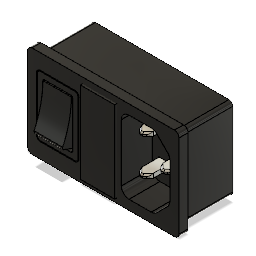
Power Receptacle (Jameco IEC-GS-1-100) v3 (Autodesk Fusion 360 design; units mm, degrees)
Autodesk Fusion 360 part; units mm, degrees
note: some values were not read from the file. Chosen so that the rebuilt part matches the saved one: which face or edge a step refers to.
sketch "Sketch1" plane through (0, 0, 0) normal (0, 0, 1) x (1, 0, 0)
  line L0 (0, 0) -> (49.9872, 0)
  line L1 (49.9872, 0) -> (49.9872, 30.48)
  line L2 (49.9872, 30.48) -> (0, 30.48)
  line L3 (0, 30.48) -> (0, 0)
  dimension "d1" = 30.48
  dimension "d2" = 49.9872
  measures "d1" distance of L0.start
  measures "d2" distance of L0.start
extrude "Extrude1" add sketch "Sketch1" against normal blind 2.9972 makes body 1
fillet "Fillet1" radius 1.4986 4 edges at (49.9872, 30.48, -1.4986) (0, 30.48, -1.4986) (0, 0, -1.4986) (49.9872, 0, -1.4986) on bodies 1
sketch "Sketch2" plane through (0, 0, -2.9972) normal (0, 0, -1) x (-1, 0, 0)
  arc A0 (-49.9872, 1.4986) -> (-48.4886, 0) centre (-48.4886, 1.4986) ccw
  line L0 (-48.4886, 0) -> (-1.4986, 0)
  arc A1 (-1.4986, 0) -> (0, 1.4986) centre (-1.4986, 1.4986) ccw
  line L1 (0, 1.4986) -> (0, 28.9814)
  arc A2 (0, 28.9814) -> (-1.4986, 30.48) centre (-1.4986, 28.9814) ccw
  line L2 (-1.4986, 30.48) -> (-48.4886, 30.48)
  arc A3 (-48.4886, 30.48) -> (-49.9872, 28.9814) centre (-48.4886, 28.9814) ccw
  line L3 (-49.9872, 28.9814) -> (-49.9872, 1.4986)
  line L4 (-24.9936, 30.48) -> (-24.9936, 0) construction
  line L5 (0, 15.24) -> (-49.9872, 15.24) construction
  line L6 (-49.9872, 30.48) -> (-49.9872, 0) construction
  line L7 (-49.9872, 0) -> (0, 0) construction
  line L8 (0, 0) -> (0, 30.48) construction
  line L9 (0, 30.48) -> (-49.9872, 30.48) construction
  line L10 (-48.2854, 1.7399) -> (-1.7018, 1.7399)
  line L11 (-1.7018, 1.7399) -> (-1.7018, 28.7401)
  line L12 (-1.7018, 28.7401) -> (-48.2854, 28.7401)
  line L13 (-48.2854, 28.7401) -> (-48.2854, 1.7399)
  line L14 (-48.2854, 28.7401) -> (-48.2854, 30.48) construction
  line L15 (-48.2854, 28.7401) -> (-49.9872, 28.7401) construction
  line L16 (-1.7018, 1.7399) -> (-1.7018, 0) construction
  line L17 (-1.7018, 1.7399) -> (0, 1.7399) construction
  dimension "d6" = 27.0002
  dimension "d7" = 46.5836
  measures "d6" distance of L7.end
  measures "d7" distance of L7.end
extrude "Extrude2" add sketch "Sketch2" along normal blind 16.4846 contours L10 L11 L12 L13 bodies 1
fillet "Fillet2" radius 1.27 4 edges at (48.2854, 28.7401, -11.2395) (1.7018, 28.7401, -11.2395) (1.7018, 1.7399, -11.2395) (48.2854, 1.7399, -11.2395) on bodies 1
sketch "Sketch3" plane through (0, 0, 0) normal (0, 0, 1) x (1, 0, 0)
  arc A0 (48.4886, 0) -> (49.9872, 1.4986) centre (48.4886, 1.4986) ccw
  line L0 (49.9872, 1.4986) -> (49.9872, 28.9814)
  arc A1 (49.9872, 28.9814) -> (48.4886, 30.48) centre (48.4886, 28.9814) ccw
  line L1 (48.4886, 30.48) -> (1.4986, 30.48)
  arc A2 (1.4986, 30.48) -> (0, 28.9814) centre (1.4986, 28.9814) ccw
  line L2 (0, 28.9814) -> (0, 1.4986)
  arc A3 (0, 1.4986) -> (1.4986, 0) centre (1.4986, 1.4986) ccw
  line L3 (1.4986, 0) -> (48.4886, 0)
  line L4 (30.9852, 5.7785) -> (30.9852, 24.7015)
  line L5 (33.5252, 27.2415) -> (40.8551, 27.2415)
  line L6 (42.6511, 26.4976) -> (46.2433, 22.9054)
  line L7 (46.9872, 21.1094) -> (46.9872, 9.3706)
  line L8 (46.2433, 7.5746) -> (42.6511, 3.9824)
  line L9 (40.8551, 3.2385) -> (33.5252, 3.2385)
  arc A4 (33.5252, 27.2415) -> (30.9852, 24.7015) centre (33.5252, 24.7015) ccw
  arc A5 (30.9852, 5.7785) -> (33.5252, 3.2385) centre (33.5252, 5.7785) ccw
  arc A6 (42.6511, 26.4976) -> (40.8551, 27.2415) centre (40.8551, 24.7015) ccw
  arc A7 (46.9872, 21.1094) -> (46.2433, 22.9054) centre (44.4472, 21.1094) ccw
  arc A8 (46.2433, 7.5746) -> (46.9872, 9.3706) centre (44.4472, 9.3706) ccw
  arc A9 (40.8551, 3.2385) -> (42.6511, 3.9824) centre (40.8551, 5.7785) ccw
  line L10 (36.1112, 3.2385) -> (36.1112, 0) construction
  line L11 (37.1901, 27.2415) -> (37.1901, 30.48) construction
  dimension "d11" = 135
  dimension "d12" = 135
  dimension "d13" = 24.003
  dimension "d14" = 16.002
  dimension "d15" = 5.08
  dimension "d16" = 2.54
  dimension "d17" = 2.54
  dimension "d18" = 3
  measures "d11" angle of L8 L9
  measures "d12" angle of L5 L6
  measures "d13" distance of origin
  measures "d14" distance of L4 L7
  measures "d16" radius of A4
  measures "d17" radius of A9
  measures "d18" distance of L0 L7
extrude "Extrude3" cut sketch "Sketch3" against normal blind 10.16 contours L4 L5 L6 L7 L8 L9 A4 A5 A6 A7 A8 A9 bodies 1
sketch "Sketch4" plane through (0, 0, 0) normal (0, 0, 1) x (1, 0, 0)
  line L0 (42.6511, 26.4976) -> (46.2433, 22.9054)
  arc A0 (46.9872, 21.1094) -> (46.2433, 22.9054) centre (44.4472, 21.1094) ccw
  line L1 (46.9872, 21.1094) -> (46.9872, 9.3706)
  arc A1 (46.2433, 7.5746) -> (46.9872, 9.3706) centre (44.4472, 9.3706) ccw
  line L2 (46.2433, 7.5746) -> (42.6511, 3.9824)
  arc A2 (40.8551, 3.2385) -> (42.6511, 3.9824) centre (40.8551, 5.7785) ccw
  line L3 (40.8551, 3.2385) -> (33.5252, 3.2385)
  arc A3 (30.9852, 5.7785) -> (33.5252, 3.2385) centre (33.5252, 5.7785) ccw
  line L4 (30.9852, 5.7785) -> (30.9852, 24.7015)
  arc A4 (33.5252, 27.2415) -> (30.9852, 24.7015) centre (33.5252, 24.7015) ccw
  line L5 (33.5252, 27.2415) -> (40.8551, 27.2415)
  arc A5 (42.6511, 26.4976) -> (40.8551, 27.2415) centre (40.8551, 24.7015) ccw
  arc A6 (48.4886, 0) -> (49.9872, 1.4986) centre (48.4886, 1.4986) ccw
  line L6 (49.9872, 1.4986) -> (49.9872, 28.9814)
  arc A7 (49.9872, 28.9814) -> (48.4886, 30.48) centre (48.4886, 28.9814) ccw
  line L7 (48.4886, 30.48) -> (1.4986, 30.48)
  arc A8 (1.4986, 30.48) -> (0, 28.9814) centre (1.4986, 28.9814) ccw
  line L8 (0, 28.9814) -> (0, 1.4986)
  arc A9 (0, 1.4986) -> (1.4986, 0) centre (1.4986, 1.4986) ccw
  line L9 (1.4986, 0) -> (48.4886, 0)
  line L10 (4.27, 5.08) -> (15.7, 5.08)
  line L11 (16.97, 6.35) -> (16.97, 24.13)
  line L12 (15.7, 25.4) -> (4.27, 25.4)
  line L13 (3, 24.13) -> (3, 6.35)
  line L14 (9.985, 25.4) -> (9.985, 30.48) construction
  line L15 (9.985, 5.08) -> (9.985, 0) construction
  arc A10 (16.97, 24.13) -> (15.7, 25.4) centre (15.7, 24.13) ccw
  arc A11 (15.7, 5.08) -> (16.97, 6.35) centre (15.7, 6.35) ccw
  arc A12 (3, 6.35) -> (4.27, 5.08) centre (4.27, 6.35) ccw
  arc A13 (4.27, 25.4) -> (3, 24.13) centre (4.27, 24.13) ccw
  dimension "d21" = 20.32
  dimension "d22" = 13.97
  dimension "d23" = 3
  dimension "d24" = 1.27
  dimension "d25" = 1.27
  measures "d23" distance of L8 L13
  measures "d24" radius of A10
  measures "d25" radius of A13
extrude "Extrude4" cut sketch "Sketch4" against normal blind 2.9972 contours L10 L11 L12 L13 A10 A11 A12 A13 bodies 1
sketch "Sketch5" plane through (0, 0, -2.9972) normal (0, 0, 1) x (1, 0, 0)
  arc A0 (4.27, 25.4) -> (3, 24.13) centre (4.27, 24.13) ccw
  line L0 (3, 24.13) -> (3, 6.35)
  arc A1 (3, 6.35) -> (4.27, 5.08) centre (4.27, 6.35) ccw
  line L1 (4.27, 5.08) -> (15.7, 5.08)
  arc A2 (15.7, 5.08) -> (16.97, 6.35) centre (15.7, 6.35) ccw
  line L2 (16.97, 6.35) -> (16.97, 24.13)
  arc A3 (16.97, 24.13) -> (15.7, 25.4) centre (15.7, 24.13) ccw
  line L3 (15.7, 25.4) -> (4.27, 25.4)
  line L4 (15.7, 6.35) -> (15.7, 24.13)
  line L5 (15.7, 24.13) -> (4.27, 24.13)
  line L6 (4.27, 24.13) -> (4.27, 6.35)
  line L7 (4.27, 6.35) -> (15.7, 6.35)
  dimension "d28" = 1.27
  measures "d28" distance of L2
extrude "Extrude5" cut sketch "Sketch5" against normal blind 50.8 contours L4 L5 L6 L7 bodies 1
sketch "Sketch6" plane through (0, 0, -2.9972) normal (0, 0, 1) x (1, 0, 0)
  line L0 (15.7, 24.13) -> (15.7, 6.35)
  line L1 (15.7, 6.35) -> (4.27, 6.35)
  line L2 (4.27, 6.35) -> (4.27, 24.13)
  line L3 (4.27, 24.13) -> (15.7, 24.13)
  arc A0 (4.27, 25.4) -> (3, 24.13) centre (4.27, 24.13) ccw
  line L4 (3, 24.13) -> (3, 6.35)
  arc A1 (3, 6.35) -> (4.27, 5.08) centre (4.27, 6.35) ccw
  line L5 (4.27, 5.08) -> (15.7, 5.08)
  arc A2 (15.7, 5.08) -> (16.97, 6.35) centre (15.7, 6.35) ccw
  line L6 (16.97, 6.35) -> (16.97, 24.13)
  arc A3 (16.97, 24.13) -> (15.7, 25.4) centre (15.7, 24.13) ccw
  line L7 (15.7, 25.4) -> (4.27, 25.4)
  line L8 (4.27, 5.334) -> (15.7, 5.334)
  arc A4 (15.7, 5.334) -> (16.716, 6.35) centre (15.7, 6.35) ccw
  line L9 (16.716, 6.35) -> (16.716, 24.13)
  arc A5 (16.716, 24.13) -> (15.7, 25.146) centre (15.7, 24.13) ccw
  line L10 (15.7, 25.146) -> (4.27, 25.146)
  arc A6 (4.27, 25.146) -> (3.254, 24.13) centre (4.27, 24.13) ccw
  line L11 (3.254, 24.13) -> (3.254, 6.35)
  arc A7 (3.254, 6.35) -> (4.27, 5.334) centre (4.27, 6.35) ccw
  line L12 (14.938, 7.112) -> (5.032, 7.112)
  line L13 (5.032, 7.112) -> (5.032, 23.368)
  line L14 (5.032, 23.368) -> (14.938, 23.368)
  line L15 (14.938, 23.368) -> (14.938, 7.112)
  dimension "d32" = 0.254
  dimension "d33" = 0.762
  measures "d32" distance of L5
  measures "d33" distance of L1
extrude "Extrude6" add sketch "Sketch6" along normal up to surface (2.9972 mm away) separate body contours L0 L1 L2 L3 | L8 A4 L9 A5 L10 A6 L11 A7 makes body 2
fillet "Fillet3" radius 0.635 4 edges at (5.032, 23.368, -1.4986) (14.938, 23.368, -1.4986) (5.032, 7.112, -1.4986) (14.938, 7.112, -1.4986) on bodies 2
sketch "Sketch7" plane through (0, 0, -2.9972) normal (0, 0, -1) x (-1, 0, 0)
  arc A0 (-14.938, 7.747) -> (-14.303, 7.112) centre (-14.303, 7.747) ccw
  line L0 (-14.938, 7.747) -> (-14.938, 22.733)
  arc A1 (-14.303, 23.368) -> (-14.938, 22.733) centre (-14.303, 22.733) ccw
  line L1 (-14.303, 23.368) -> (-5.667, 23.368)
  arc A2 (-5.032, 22.733) -> (-5.667, 23.368) centre (-5.667, 22.733) ccw
  line L2 (-5.032, 22.733) -> (-5.032, 7.747)
  arc A3 (-5.667, 7.112) -> (-5.032, 7.747) centre (-5.667, 7.747) ccw
  line L3 (-5.667, 7.112) -> (-14.303, 7.112)
  arc A4 (-4.27, 5.334) -> (-3.254, 6.35) centre (-4.27, 6.35) ccw
  line L4 (-3.254, 6.35) -> (-3.254, 24.13)
  arc A5 (-3.254, 24.13) -> (-4.27, 25.146) centre (-4.27, 24.13) ccw
  line L5 (-4.27, 25.146) -> (-15.7, 25.146)
  arc A6 (-15.7, 25.146) -> (-16.716, 24.13) centre (-15.7, 24.13) ccw
  line L6 (-16.716, 24.13) -> (-16.716, 6.35)
  arc A7 (-16.716, 6.35) -> (-15.7, 5.334) centre (-15.7, 6.35) ccw
  line L7 (-15.7, 5.334) -> (-4.27, 5.334)
  line L8 (-15.1788, 23.6625) -> (-4.7856, 23.6625)
  line L9 (-4.7856, 23.6625) -> (-4.7856, 6.7161)
  line L10 (-4.7856, 6.7161) -> (-15.1788, 6.7161)
  line L11 (-15.1788, 6.7161) -> (-15.1788, 23.6625)
extrude "Extrude7" add sketch "Sketch7" along normal blind 11.43 contours A0 L0 A1 L1 A2 L2 A3 L3 | L8 L9 L10 L11 bodies 2
sketch "Sketch8" plane through (0, 0, -2.9972) normal (0, 0, 1) x (1, 0, 0)
  arc A0 (14.938, 22.733) -> (14.303, 23.368) centre (14.303, 22.733) ccw
  line L0 (14.303, 23.368) -> (5.667, 23.368)
  arc A1 (5.667, 23.368) -> (5.032, 22.733) centre (5.667, 22.733) ccw
  line L1 (5.032, 22.733) -> (5.032, 7.747)
  arc A2 (5.032, 7.747) -> (5.667, 7.112) centre (5.667, 7.747) ccw
  line L2 (5.667, 7.112) -> (14.303, 7.112)
  arc A3 (14.303, 7.112) -> (14.938, 7.747) centre (14.303, 7.747) ccw
  line L3 (14.938, 7.747) -> (14.938, 22.733)
  line L4 (14.684, 7.747) -> (14.684, 22.733)
  arc A4 (14.684, 22.733) -> (14.303, 23.114) centre (14.303, 22.733) ccw
  line L5 (14.303, 23.114) -> (5.667, 23.114)
  arc A5 (5.667, 23.114) -> (5.286, 22.733) centre (5.667, 22.733) ccw
  line L6 (5.286, 22.733) -> (5.286, 7.747)
  arc A6 (5.286, 7.747) -> (5.667, 7.366) centre (5.667, 7.747) ccw
  line L7 (5.667, 7.366) -> (14.303, 7.366)
  arc A7 (14.303, 7.366) -> (14.684, 7.747) centre (14.303, 7.747) ccw
  dimension "d39" = 0.254
  measures "d39" distance of L3
extrude "Extrude8" add sketch "Sketch8" along normal blind 6.35 separate body contours L4 A4 L5 A5 L6 A6 L7 A7 makes body 3
sketch "Sketch9" plane through (5.286, 0, 0) normal (-1, 0, 0) x (0, 0, 1)
  line L0 (-2.9972, 7.747) -> (3.3528, 7.747)
  line L1 (3.3528, 7.747) -> (3.3528, 22.733)
  line L2 (3.3528, 22.733) -> (-2.9972, 22.733)
  line L3 (-2.9972, 7.2231) -> (3.3528, 9.5788)
  arc A0 (0.1778, 23.4401) -> (3.3528, 9.5788) centre (31.7454, 23.3766) ccw
  line L4 (-2.9972, 7.2231) -> (-2.9972, -1.1091)
  line L5 (-2.9972, -1.1091) -> (15.3397, -2.5698)
  line L6 (15.3397, -2.5698) -> (9.4997, 23.1267)
  line L7 (9.4997, 23.1267) -> (0.1778, 23.4401)
  line L8 (-2.9972, 22.733) -> (-2.9972, 7.747)
extrude "Extrude9" cut sketch "Sketch9" against normal blind 20.32 contours L0 L1 L3 | L0 L1 L2 L3 A0 L4 L5 L6 L7 | L1 L2 A0 bodies 3
fillet "Fillet4" radius 0.635 1 edges at (9.985, 9.5788, 3.3528) on bodies 3
sketch "Sketch10" plane through (0, 0, 0) normal (0, 0, 1) x (1, 0, 0)
  line L0 (3, 6.35) -> (3, 24.13)
  arc A0 (4.27, 25.4) -> (3, 24.13) centre (4.27, 24.13) ccw
  line L1 (4.27, 25.4) -> (15.7, 25.4)
  arc A1 (16.97, 24.13) -> (15.7, 25.4) centre (15.7, 24.13) ccw
  line L2 (16.97, 24.13) -> (16.97, 6.35)
  arc A2 (15.7, 5.08) -> (16.97, 6.35) centre (15.7, 6.35) ccw
  line L3 (15.7, 5.08) -> (4.27, 5.08)
  arc A3 (3, 6.35) -> (4.27, 5.08) centre (4.27, 6.35) ccw
  line L4 (42.6511, 26.4976) -> (46.2433, 22.9054)
  arc A4 (46.9872, 21.1094) -> (46.2433, 22.9054) centre (44.4472, 21.1094) ccw
  line L5 (46.9872, 21.1094) -> (46.9872, 9.3706)
  arc A5 (46.2433, 7.5746) -> (46.9872, 9.3706) centre (44.4472, 9.3706) ccw
  line L6 (46.2433, 7.5746) -> (42.6511, 3.9824)
  arc A6 (40.8551, 3.2385) -> (42.6511, 3.9824) centre (40.8551, 5.7785) ccw
  line L7 (40.8551, 3.2385) -> (33.5252, 3.2385)
  arc A7 (30.9852, 5.7785) -> (33.5252, 3.2385) centre (33.5252, 5.7785) ccw
  line L8 (30.9852, 5.7785) -> (30.9852, 24.7015)
  arc A8 (33.5252, 27.2415) -> (30.9852, 24.7015) centre (33.5252, 24.7015) ccw
  line L9 (33.5252, 27.2415) -> (40.8551, 27.2415)
  arc A9 (42.6511, 26.4976) -> (40.8551, 27.2415) centre (40.8551, 24.7015) ccw
  arc A10 (48.4886, 0) -> (49.9872, 1.4986) centre (48.4886, 1.4986) ccw
  line L10 (49.9872, 1.4986) -> (49.9872, 28.9814)
  arc A11 (49.9872, 28.9814) -> (48.4886, 30.48) centre (48.4886, 28.9814) ccw
  line L11 (48.4886, 30.48) -> (1.4986, 30.48)
  arc A12 (1.4986, 30.48) -> (0, 28.9814) centre (1.4986, 28.9814) ccw
  line L12 (0, 28.9814) -> (0, 1.4986)
  arc A13 (0, 1.4986) -> (1.4986, 0) centre (1.4986, 1.4986) ccw
  line L13 (1.4986, 0) -> (48.4886, 0)
  line L14 (19.5925, 27.5743) -> (28.391, 27.5743)
  line L15 (28.391, 27.5743) -> (28.391, 2.7579)
  line L16 (28.391, 2.7579) -> (19.5925, 2.7579)
  line L17 (19.5925, 2.7579) -> (19.5925, 27.5743)
extrude "Extrude10" cut sketch "Sketch10" against normal blind 7.62 contours L14 L15 L16 L17 bodies 1
sketch "Sketch11" plane through (0, 0, 0) normal (0, 0, 1) x (1, 0, 0)
  line L0 (28.391, 27.5743) -> (28.391, 2.7579)
  line L1 (28.391, 2.7579) -> (19.5925, 2.7579)
  line L2 (19.5925, 2.7579) -> (19.5925, 27.5743)
  line L3 (19.5925, 27.5743) -> (28.391, 27.5743)
  line L4 (3, 6.35) -> (3, 24.13)
  arc A0 (4.27, 25.4) -> (3, 24.13) centre (4.27, 24.13) ccw
  line L5 (4.27, 25.4) -> (15.7, 25.4)
  arc A1 (16.97, 24.13) -> (15.7, 25.4) centre (15.7, 24.13) ccw
  line L6 (16.97, 24.13) -> (16.97, 6.35)
  arc A2 (15.7, 5.08) -> (16.97, 6.35) centre (15.7, 6.35) ccw
  line L7 (15.7, 5.08) -> (4.27, 5.08)
  arc A3 (3, 6.35) -> (4.27, 5.08) centre (4.27, 6.35) ccw
  line L8 (42.6511, 26.4976) -> (46.2433, 22.9054)
  arc A4 (46.9872, 21.1094) -> (46.2433, 22.9054) centre (44.4472, 21.1094) ccw
  line L9 (46.9872, 21.1094) -> (46.9872, 9.3706)
  arc A5 (46.2433, 7.5746) -> (46.9872, 9.3706) centre (44.4472, 9.3706) ccw
  line L10 (46.2433, 7.5746) -> (42.6511, 3.9824)
  arc A6 (40.8551, 3.2385) -> (42.6511, 3.9824) centre (40.8551, 5.7785) ccw
  line L11 (40.8551, 3.2385) -> (33.5252, 3.2385)
  arc A7 (30.9852, 5.7785) -> (33.5252, 3.2385) centre (33.5252, 5.7785) ccw
  line L12 (30.9852, 5.7785) -> (30.9852, 24.7015)
  arc A8 (33.5252, 27.2415) -> (30.9852, 24.7015) centre (33.5252, 24.7015) ccw
  line L13 (33.5252, 27.2415) -> (40.8551, 27.2415)
  arc A9 (42.6511, 26.4976) -> (40.8551, 27.2415) centre (40.8551, 24.7015) ccw
  arc A10 (48.4886, 0) -> (49.9872, 1.4986) centre (48.4886, 1.4986) ccw
  line L14 (49.9872, 1.4986) -> (49.9872, 28.9814)
  arc A11 (49.9872, 28.9814) -> (48.4886, 30.48) centre (48.4886, 28.9814) ccw
  line L15 (48.4886, 30.48) -> (1.4986, 30.48)
  arc A12 (1.4986, 30.48) -> (0, 28.9814) centre (1.4986, 28.9814) ccw
  line L16 (0, 28.9814) -> (0, 1.4986)
  arc A13 (0, 1.4986) -> (1.4986, 0) centre (1.4986, 1.4986) ccw
  line L17 (1.4986, 0) -> (48.4886, 0)
  line L18 (18.1348, 28.4955) -> (29.415, 28.4955)
  line L19 (29.415, 28.4955) -> (29.415, 1.5359)
  line L20 (29.415, 1.5359) -> (18.1348, 1.5359)
  line L21 (18.1348, 1.5359) -> (18.1348, 28.4955)
extrude "Extrude11" add sketch "Sketch11" along normal blind 0.635 and the other way blind 0.254 separate body contours L0 L1 L2 L3 | L18 L19 L20 L21 makes body 4
shell "Shell2" thickness 2.54 removed faces 1 at (36.5769, 18.2033, -19.4818) on bodies 1
sketch "Sketch12" plane through (0, 0, -10.16) normal (0, 0, 1) x (1, 0, 0)
  line L0 (33.5252, 3.2385) -> (40.8551, 3.2385)
  arc A0 (40.8551, 3.2385) -> (42.6511, 3.9824) centre (40.8551, 5.7785) ccw
  line L1 (42.6511, 3.9824) -> (46.2433, 7.5746)
  arc A1 (46.2433, 7.5746) -> (46.9872, 9.3706) centre (44.4472, 9.3706) ccw
  line L2 (46.9872, 9.3706) -> (46.9872, 21.1094)
  arc A2 (46.9872, 21.1094) -> (46.2433, 22.9054) centre (44.4472, 21.1094) ccw
  line L3 (46.2433, 22.9054) -> (42.6511, 26.4976)
  arc A3 (42.6511, 26.4976) -> (40.8551, 27.2415) centre (40.8551, 24.7015) ccw
  line L4 (40.8551, 27.2415) -> (33.5252, 27.2415)
  arc A4 (33.5252, 27.2415) -> (30.9852, 24.7015) centre (33.5252, 24.7015) ccw
  line L5 (30.9852, 24.7015) -> (30.9852, 5.7785)
  arc A5 (30.9852, 5.7785) -> (33.5252, 3.2385) centre (33.5252, 5.7785) ccw
  line L6 (46.9872, 15.24) -> (30.9852, 15.24) construction
  line L7 (38.9862, 15.24) -> (38.9862, 27.2415) construction
  line L8 (38.9862, 15.24) -> (38.9862, 3.2385) construction
  line L9 (38.9862, 21.2407) -> (30.9852, 21.2407) construction
  line L10 (38.9862, 9.2393) -> (30.9852, 9.2393) construction
  line L11 (33.0599, 22.0725) -> (36.9115, 22.0725)
  line L12 (36.9115, 22.0725) -> (36.9115, 20.409)
  line L13 (36.9115, 20.409) -> (33.0599, 20.409)
  line L14 (33.0599, 20.409) -> (33.0599, 22.0725)
  line L15 (33.0599, 22.0725) -> (36.9115, 20.409) construction
  line L16 (36.9115, 22.0725) -> (33.0599, 20.409) construction
  line L17 (41.3317, 16.0718) -> (45.1833, 16.0718)
  line L18 (45.1833, 16.0718) -> (45.1833, 14.4082)
  line L19 (45.1833, 14.4082) -> (41.3317, 14.4082)
  line L20 (41.3317, 14.4082) -> (41.3317, 16.0718)
  line L21 (41.3317, 16.0718) -> (45.1833, 14.4082) construction
  line L22 (45.1833, 16.0718) -> (41.3317, 14.4082) construction
  line L23 (33.0599, 8.4075) -> (36.9115, 8.4075)
  line L24 (36.9115, 8.4075) -> (36.9115, 10.071)
  line L25 (36.9115, 10.071) -> (33.0599, 10.071)
  line L26 (33.0599, 10.071) -> (33.0599, 8.4075)
extrude "Extrude12" cut sketch "Sketch12" against normal blind 15.24 contours L11 L12 L13 L14 | L17 L18 L19 L20 | L23 L24 L25 L26 bodies 1
sketch "Sketch13" plane through (0, 0, -10.16) normal (0, 0, 1) x (1, 0, 0)
  line L0 (36.9115, 22.0725) -> (36.9115, 20.409)
  line L1 (36.9115, 20.409) -> (33.0599, 20.409)
  line L2 (33.0599, 20.409) -> (33.0599, 22.0725)
  line L3 (33.0599, 22.0725) -> (36.9115, 22.0725)
  line L4 (45.1833, 16.0718) -> (45.1833, 14.4082)
  line L5 (45.1833, 14.4082) -> (41.3317, 14.4082)
  line L6 (41.3317, 14.4082) -> (41.3317, 16.0718)
  line L7 (41.3317, 16.0718) -> (45.1833, 16.0718)
  line L8 (36.9115, 8.4075) -> (33.0599, 8.4075)
  line L9 (33.0599, 8.4075) -> (33.0599, 10.071)
  line L10 (33.0599, 10.071) -> (36.9115, 10.071)
  line L11 (36.9115, 10.071) -> (36.9115, 8.4075)
  line L12 (33.5252, 3.2385) -> (40.8551, 3.2385)
  arc A0 (40.8551, 3.2385) -> (42.6511, 3.9824) centre (40.8551, 5.7785) ccw
  line L13 (42.6511, 3.9824) -> (46.2433, 7.5746)
  arc A1 (46.2433, 7.5746) -> (46.9872, 9.3706) centre (44.4472, 9.3706) ccw
  line L14 (46.9872, 9.3706) -> (46.9872, 21.1094)
  arc A2 (46.9872, 21.1094) -> (46.2433, 22.9054) centre (44.4472, 21.1094) ccw
  line L15 (46.2433, 22.9054) -> (42.6511, 26.4976)
  arc A3 (42.6511, 26.4976) -> (40.8551, 27.2415) centre (40.8551, 24.7015) ccw
  line L16 (40.8551, 27.2415) -> (33.5252, 27.2415)
  arc A4 (33.5252, 27.2415) -> (30.9852, 24.7015) centre (33.5252, 24.7015) ccw
  line L17 (30.9852, 24.7015) -> (30.9852, 5.7785)
  arc A5 (30.9852, 5.7785) -> (33.5252, 3.2385) centre (33.5252, 5.7785) ccw
  line L18 (33.1869, 21.9455) -> (36.7845, 21.9455)
  line L19 (36.7845, 21.9455) -> (36.7845, 20.536)
  line L20 (36.7845, 20.536) -> (33.1869, 20.536)
  line L21 (33.1869, 20.536) -> (33.1869, 21.9455)
  line L22 (45.0563, 14.5352) -> (41.4587, 14.5352)
  line L23 (41.4587, 14.5352) -> (41.4587, 15.9448)
  line L24 (41.4587, 15.9448) -> (45.0563, 15.9448)
  line L25 (45.0563, 15.9448) -> (45.0563, 14.5352)
  line L26 (36.7845, 8.5345) -> (33.1869, 8.5345)
  line L27 (33.1869, 8.5345) -> (33.1869, 9.944)
  line L28 (33.1869, 9.944) -> (36.7845, 9.944)
  line L29 (36.7845, 9.944) -> (36.7845, 8.5345)
  dimension "d54" = 0.127
  dimension "d55" = 0.127
  dimension "d56" = 0.127
  measures "d55" distance of L5
  measures "d56" distance of L8
extrude "Extrude13" add sketch "Sketch13" along normal blind 8.89 and the other way up to surface (2.54 mm away) separate body contours L22 L23 L24 L25 makes body 5
extrude "Extrude14" add sketch "Sketch13" along normal up to surface (7.62 mm away) and the other way up to surface (2.54 mm away) separate body contours L18 L19 L20 L21 | L26 L27 L28 L29 makes body 6 at (34.3861, 8.5345, -5.9267) makes body 7 at (35.5853, 21.9455, -5.9267)
chamfer "Chamfer1" distance 1.27 angle 45 6 edges at (36.7845, 9.2393, -2.54) (33.1869, 9.2393, -2.54) (36.7845, 21.2407, -2.54) (33.1869, 21.2407, -2.54) (45.0563, 15.24, -1.27) (41.4587, 15.24, -1.27) on bodies 5 6 7
chamfer "Chamfer2" distance 0.508 angle 45 18 edges at (36.1495, 9.944, -3.175) (34.9857, 9.944, -2.54) (33.8219, 9.944, -3.175) (33.8219, 8.5345, -3.175) (34.9857, 8.5345, -2.54) (36.1495, 8.5345, -3.175) (36.1495, 20.536, -3.175) (34.9857, 20.536, -2.54) (33.8219, 20.536, -3.175) (33.8219, 21.9455, -3.175) (34.9857, 21.9455, -2.54) (36.1495, 21.9455, -3.175) (44.4213, 14.5352, -1.905) (43.2575, 14.5352, -1.27) (42.0937, 14.5352, -1.905) (42.0937, 15.9448, -1.905) (43.2575, 15.9448, -1.27) (44.4213, 15.9448, -1.905) on bodies 5 6 7
fillet "Fillet5" radius 2.286 6 edges at (41.4587, 15.24, -2.54) (45.0563, 15.24, -2.54) (33.1869, 9.2393, -3.81) (36.7845, 9.2393, -3.81) (36.7845, 21.2407, -3.81) (33.1869, 21.2407, -3.81) on bodies 5 6 7
equation "d8 = 0.767 in - 0.118 in"
